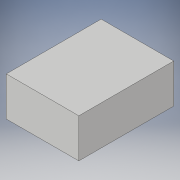
# Autodesk Inventor part: AC2DC_real
Saved by Autodesk Inventor 2018 (Build 220112000, 112)
## iProperties
Created: 2018-02-10
Part Number: AC2DC_real
Material: Generic
Document SubType Name: Modeling
Designer: artur
Density: 1 g/cm^3
Appearance: Default
Author: artur
Autodesk Inventor part; units mm, degrees
ref_plane "YZ Plane" through (0, 0, 0) normal (1, 0, 0) x (0, 1, 0)
ref_plane "XZ Plane" through (0, 0, 0) normal (0, 1, 0) x (-1, 0, 0)
ref_plane "XY Plane" through (0, 0, 0) normal (0, 0, 1) x (1, 0, 0)
sketch "Sketch1" plane through (0, 0, 0) normal (0, 1, 0) x (-1, 0, 0)
  line L0 (0, 0) -> (33.02, 0)
  line L1 (33.02, 0) -> (33.02, -43.18)
  line L2 (33.02, -43.18) -> (0, -43.18)
  line L3 (0, -43.18) -> (0, 0)
  dimension "d0" = 43.18
  dimension "d1" = 33.02
  constraints: 8 end point, 2 parallel, 1 horizontal, 1 perpendicular
  measures "d0" distance of L0.end L1.end
  measures "d1" distance of L1.end L2.end
extrude "Extrusion1" add sketch "Sketch1" along normal blind 17.78
body "Solid1"
